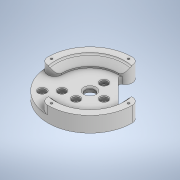
# Autodesk Inventor part: Union_fija_lazy_susan
Saved by Autodesk Inventor 2021 (Build 250183000, 183)
## iProperties
Created: 2021-01-16
Part Number: Union_fija_lazy_susan
Material: Generic
Document SubType Name: Modeling
Designer: jorge
Density: 1 g/cm^3
Appearance: Default
Author: jorge
Autodesk Inventor part; units mm, degrees
ref_plane "YZ Plane" through (0, 0, 0) normal (1, 0, 0) x (0, 1, 0)
ref_plane "XZ Plane" through (0, 0, 0) normal (0, 1, 0) x (-1, 0, 0)
ref_plane "XY Plane" through (0, 0, 0) normal (0, 0, 1) x (1, 0, 0)
sketch "Sketch1" plane through (0, 0, 0) normal (0, 1, 0) x (-1, 0, 0)
  circle A0 centre (0, 0) radius 60
  dimension "d0" = 120
  constraints: 1 centre point, 1 coincident
  measures "d0" diameter of A0
extrude "Extrusion1" add sketch "Sketch1" along normal blind 10
sketch "Sketch2" plane through (0, 10, 0) normal (0, 1, 0) x (1, 0, 0)
  circle A0 centre (0, 0) radius 60
  circle A1 centre (0, 0) radius 60 projected
  circle A2 centre (0, 0) radius 40
  dimension "d3" = 80
  constraints: 2 centre point, 2 coincident, 1 concentric
  measures "d3" diameter of A2
extrude "Extrusion2" add sketch "Sketch2" along normal blind 10
sketch "Sketch3" plane through (0, 20, 0) normal (0, 1, 0) x (1, 0, 0)
  circle A0 centre (0, 0) radius 60
  circle A1 centre (0, 0) radius 60 projected
  circle A2 centre (0, 0) radius 50
  dimension "d6" = 100
  constraints: 2 centre point, 2 coincident, 1 concentric
  measures "d6" diameter of A2
extrude "Extrusion3" add sketch "Sketch3" along normal blind 2
fillet "Fillet1" radius 2 1 edges at (-50, 20, 0)
chamfer "Chamfer1" distance 8 angle 45 1 edges at (-40, 20, 0)
sketch "Sketch4" plane through (0, 22, 0) normal (0, 1, 0) x (1, 0, 0)
  circle A0 centre (0, -55) radius 1.55
  circle A1 centre (-55, 0) radius 1.55
  circle A2 centre (0, 55) radius 1.55
  circle A3 centre (55, 0) radius 1.55
  point P0 (0, 0)
  dimension "d13" = 3.1
  dimension "d14" = 3.1
  dimension "d15" = 3.1
  dimension "d16" = 3.1
  dimension "d17" = 0
  dimension "d18" = 0
  dimension "d19" = 0
  dimension "d20" = 55
  dimension "d21" = 55
  dimension "d22" = 55
  dimension "d23" = 55
  dimension "d24" = 0
  constraints: 4 centre point
  measures "d13" diameter of A0
  measures "d14" diameter of A1
  measures "d15" diameter of A2
  measures "d16" diameter of A3
  measures "d17" horizontal distance of point (0, 0) A0.centre
  measures "d18" vertical distance of point (0, 0) A1.centre
  measures "d19" horizontal distance of point (0, 0) A2.centre
  measures "d20" distance of point (0, 0) A2.centre
  measures "d21" distance of A1.centre point (0, 0)
  measures "d22" distance of point (0, 0) A0.centre
  measures "d23" distance of A3.centre point (0, 0)
  measures "d24" vertical distance of point (0, 0) A3.centre
extrude "Extrusion4" cut sketch "Sketch4" against normal up to surface (22 mm away)
sketch "Sketch5" plane through (0, 0, 0) normal (0, -1, 0) x (1, 0, 0)
  circle A0 centre (55, 0) radius 1.55
  line L0 (55, -3.175426) -> (52.25, -1.587713)
  line L1 (52.25, -1.587713) -> (52.25, 1.587713)
  line L2 (52.25, 1.587713) -> (55, 3.175426)
  line L3 (55, 3.175426) -> (57.75, 1.587713)
  line L4 (57.75, 1.587713) -> (57.75, -1.587713)
  line L5 (57.75, -1.587713) -> (55, -3.175426)
  circle A1 centre (0, -55) radius 1.55
  line L6 (3.175426, -55) -> (1.587713, -57.75)
  line L7 (1.587713, -57.75) -> (-1.587713, -57.75)
  line L8 (-1.587713, -57.75) -> (-3.175426, -55)
  line L9 (-3.175426, -55) -> (-1.587713, -52.25)
  line L10 (-1.587713, -52.25) -> (1.587713, -52.25)
  line L11 (1.587713, -52.25) -> (3.175426, -55)
  circle A2 centre (-55, 0) radius 1.55
  line L12 (-52.25, 1.587713) -> (-52.25, -1.587713)
  line L13 (-52.25, -1.587713) -> (-55, -3.175426)
  line L14 (-55, -3.175426) -> (-57.75, -1.587713)
  line L15 (-57.75, -1.587713) -> (-57.75, 1.587713)
  line L16 (-57.75, 1.587713) -> (-55, 3.175426)
  line L17 (-55, 3.175426) -> (-52.25, 1.587713)
  circle A3 centre (0, 55) radius 1.55
  line L18 (-3.175426, 55) -> (-1.587713, 57.75)
  line L19 (-1.587713, 57.75) -> (1.587713, 57.75)
  line L20 (1.587713, 57.75) -> (3.175426, 55)
  line L21 (3.175426, 55) -> (1.587713, 52.25)
  line L22 (1.587713, 52.25) -> (-1.587713, 52.25)
  line L23 (-1.587713, 52.25) -> (-3.175426, 55)
  line L24 (0, -84) -> (0, 84)
  line L25 (-84, 0) -> (84, 0)
  point P0 (0, 0)
  dimension "d27" = 5.5
  dimension "d28" = 5.5
  dimension "d29" = 5.5
  dimension "d30" = 5.5
  constraints: 48 end point, 4 coincident, 4 parallel, 52 other
  measures "d27" distance between parallel lines of L20 L23
  measures "d28" distance between parallel lines of L2 L5
  measures "d29" distance between parallel lines of L10 L7
  measures "d30" distance between parallel lines of L16 L13
extrude "Extrusion5" cut sketch "Sketch5" against normal blind 5
sketch "Sketch6" plane through (0, 10, 0) normal (0, 1, 0) x (1, 0, 0)
  line L0 (60.104076, 24.748737) -> (-24.748737, -60.104076)
  line L1 (-24.748737, -60.104076) -> (-60.104076, -24.748737)
  line L2 (-60.104076, -24.748737) -> (24.748737, 60.104076)
  line L3 (24.748737, 60.104076) -> (60.104076, 24.748737)
  circle A0 centre (0, 0) radius 60
  line L4 (-85.902365, 0) -> (85.902365, 0)
  dimension "d33" = 25
  dimension "d34" = 25
  dimension "d35" = 45
  constraints: 8 end point, 2 parallel, 2 tangent, 1 perpendicular
  measures "d33" distance from line of L2 point (0, 0)
  measures "d34" distance from line of L0 point (0, 0)
  measures "d35" angle of L4 L0
extrude "Extrusion6" cut sketch "Sketch6" along normal blind 25 contours L0 A0 L3 | L0 L4 L2 A0 | A0 L2 L3 | L0 A0 L2 L4 | L0 L1 A0 | L1 L2 A0
fillet "Fillet2" radius 10 8 edges at (39.7571, 11, -4.4017) (56.2458, 16, -20.8905) (-4.4017, 11, 39.7571) (-20.8905, 16, 56.2458) (4.4017, 11, -39.7571) (20.8905, 16, -56.2458) (-56.2458, 16, 20.8905) (-39.7571, 11, 4.4017)
sketch "Sketch7" plane through (0, 0, 0) normal (0, -1, 0) x (1, 0, 0)
  circle A0 centre (0, 0) radius 11.2
  dimension "d39" = 22.4
  constraints: 1 centre point, 1 coincident
  measures "d39" diameter of A0
extrude "Extrusion7" cut sketch "Sketch7" against normal blind 7
sketch "Sketch8" plane through (0, 7, 0) normal (0, -1, 0) x (1, 0, 0)
  circle A0 centre (0, 0) radius 7
  dimension "d42" = 14
  constraints: 1 centre point, 1 coincident
  measures "d42" diameter of A0
extrude "Extrusion8" cut sketch "Sketch8" against normal up to surface (3 mm away)
chamfer "Chamfer2" distance 2 angle 45 1 edges at (-7, 10, 0)
sketch "Sketch10" plane through (0, 10, 0) normal (0, 1, 0) x (1, 0, 0)
  circle A0 centre (0, 20) radius 2.05
  circle A1 centre (20, 0) radius 2.05
  circle A2 centre (0, -20) radius 2.05
  circle A3 centre (-20, 0) radius 2.05
  circle A4 centre (-20, -20) radius 2.05
  circle A5 centre (-34.142136, -34.142136) radius 2.05
  line L0 (0, 0) -> (-34.142136, -34.142136)
  dimension "d48" = 4.1
  dimension "d49" = 4.1
  dimension "d50" = 4.1
  dimension "d51" = 4.1
  dimension "d52" = 0
  dimension "d53" = 0
  dimension "d54" = 0
  dimension "d55" = 0
  dimension "d56" = 40
  dimension "d57" = 20
  dimension "d58" = 40
  dimension "d59" = 20
  dimension "d62" = 4.1
  dimension "d63" = 20
  dimension "d64" = 20
  dimension "d65" = 4.1
  dimension "d66" = 20
  constraints: 6 centre point, 2 end point, 1 point on line
  measures "d48" diameter of A0
  measures "d49" diameter of A1
  measures "d50" diameter of A2
  measures "d51" diameter of A3
  measures "d52" horizontal distance of A0.centre L0.start
  measures "d53" vertical distance of A3.centre L0.start
  measures "d54" horizontal distance of L0.start A2.centre
  measures "d55" vertical distance of L0.start A1.centre
  measures "d56" distance of A3.centre A1.centre
  measures "d57" distance of A1.centre L0.start
  measures "d58" distance of A0.centre A2.centre
  measures "d59" distance of L0.start A2.centre
  measures "d62" diameter of A4
  measures "d63" distance of A4.centre A2.centre
  measures "d64" distance of A3.centre A4.centre
  measures "d65" diameter of A5
  measures "d66" distance of L0.end A4.centre
extrude "Extrusion9" cut sketch "Sketch10" against normal up to surface (10 mm away) contours A0 | A1 | A2 | A4 L0 | L0 A4 | A5
sketch "Sketch12" plane through (0, 10, 0) normal (0, 1, 0) x (1, 0, 0)
  arc A0 (59.997, 0.60003) -> (48.898046, 10.439401) centre (49.9975, 0.500025) ccw
  arc A1 (59.997, 0.60003) -> (48.898046, 10.439401) centre (49.9975, 0.500025) ccw
  arc A2 (59.997, 0.60003) -> (39.998, 0.40002) centre (49.9975, 0.500025) ccw
  arc A3 (48.898046, 10.439401) -> (39.998, 0.40002) centre (49.9975, 0.500025) ccw
  arc A4 (0.40002, 39.998) -> (0.60003, 59.997) centre (0.500025, 49.9975) ccw
  arc A5 (0.40002, 39.998) -> (0.60003, 59.997) centre (0.500025, 49.9975) ccw
  arc A6 (0.40002, 39.998) -> (-39.998, -0.40002) centre (0, 0) ccw
  line L0 (39.998, 0.40002) -> (0.40002, 39.998)
  arc A7 (59.997, 0.60003) -> (0.60003, 59.997) centre (0, 0) ccw
  arc A8 (59.997, 0.60003) -> (0.60003, 59.997) centre (0, 0) ccw
  dimension "d67" = 10
  dimension "d68" = 10
  dimension "d69" = 10
  dimension "d70" = 60
  constraints: 8 point on circle, 4 centre point, 2 end point
  measures "d67" radius of A1
  measures "d68" radius of A3
  measures "d69" radius of A5
  measures "d70" radius of A8
extrude "Extrusion10" cut sketch "Sketch12" against normal up to surface (10 mm away)
fillet "Fillet3" radius 3 2 edges at (39.998, 5, -0.4) (0.4, 5, -39.998)
sketch "Sketch13" plane through (0, 10, 0) normal (0, 1, 0) x (1, 0, 0)
  circle A0 centre (-34.142136, -34.142136) radius 2.05
  circle A1 centre (-34.142136, -34.142136) radius 5
  circle A2 centre (-20, -20) radius 2.05
  circle A3 centre (-20, -20) radius 5
  circle A4 centre (0, -20) radius 2.05
  circle A5 centre (0, -20) radius 5
  circle A6 centre (0, 20) radius 2.05
  circle A7 centre (0, 20) radius 5
  circle A8 centre (20, 0) radius 2.05
  circle A9 centre (20, 0) radius 5
  point P0 (0, 0)
  dimension "d74" = 10
  dimension "d75" = 10
  dimension "d76" = 10
  dimension "d77" = 10
  dimension "d78" = 10
  constraints: 5 centre point, 5 coincident
  measures "d74" diameter of A1
  measures "d75" diameter of A3
  measures "d76" diameter of A5
  measures "d77" diameter of A7
  measures "d78" diameter of A9
extrude "Extrusion11" cut sketch "Sketch13" against normal blind 5 contours A0 | A1 | A2 | A3 | A4 | A5 | A6 | A7 | A8 | A9
chamfer "Chamfer3" distance 1 angle 45 5 edges at (-5, 10, -20) (-25, 10, 20) (-39.1421, 10, 34.1421) (-5, 10, 20) (15, 10, 0)
equation "\"d36\" = d34"
body "Solid1"
